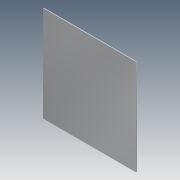
# Autodesk Inventor part: base plate
Saved by Autodesk Inventor 2014 (Build 180170000, 170)
## iProperties
Created: 2016-01-12
Part Number: base plate
Material: Aluminum 6061-AHC
Document SubType Name: Modeling
Designer: Paul
Mass: 2198.24 g
Surface Area: 5177.25 cm^2
Volume: 811.16 cm^3
Density: 2.71 g/cm^3
Appearance: Machined - Aluminum
Author: Paul
Autodesk Inventor part; units mm, degrees
ref_plane "YZ Plane" through (0, 0, 0) normal (1, 0, 0) x (0, 1, 0)
ref_plane "XZ Plane" through (0, 0, 0) normal (0, 1, 0) x (-1, 0, 0)
ref_plane "XY Plane" through (0, 0, 0) normal (0, 0, 1) x (1, 0, 0)
sketch "Sketch1" plane through (0, 0, 0) normal (0, 0, 1) x (1, 0, 0)
  line L0 (0, 0) -> (355.6, 0)
  line L1 (355.6, 0) -> (355.6, 365.76)
  line L2 (355.6, 365.76) -> (0, 365.76)
  line L3 (0, 365.76) -> (0, 0)
  dimension "d0" = 355.6
  dimension "d1" = 365.76
  constraints: 8 end point, 2 parallel, 1 horizontal, 1 perpendicular
  measures "d0" distance of L2.end L1.end
  measures "d1" distance of L1.end L0.end
extrude "Extrusion1" add sketch "Sketch1" along normal blind 3.175
body "Solid1"
